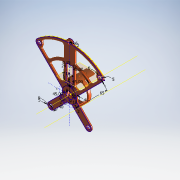
# Autodesk Inventor part: Pok Yaw Motor Face Mount
Saved by Autodesk Inventor 2018.2 (Build 222227000, 227)
## iProperties
Created: 2018-02-07
Part Number: Pok Yaw Motor Face Mount
Material: ABS Plastic
Document SubType Name: Modeling
Designer: Moochster
Density: 1.06 g/cm^3
Appearance: Smooth - Light Orange
Author: Moochster
Autodesk Inventor part; units mm, degrees
ref_plane "XZ Plane" through (0, 0, 0) normal (0, 1, 0) x (-1, 0, 0)
sketch "Sketch1" plane through (0, 0, 0) normal (0, 1, 0) x (-1, 0, 0)
  circle A0 centre (0, 0) radius 5 construction
  circle A1 centre (0, 0) radius 5.15
  circle A2 centre (8, 0) radius 1.25
  circle A3 centre (-8, 0) radius 1.25
  arc A4 (10.836268, 1.890843) -> (10.463737, 3.392669) centre (0, 0) ccw
  circle A5 centre (0, 0) radius 15 construction
  arc A6 (6.505618, 15.705952) -> (-6.505618, 15.705952) centre (0, 0) ccw
  arc A7 (5.740251, 13.858193) -> (-5.740251, 13.858193) centre (0, 0) ccw
  line L0 (6.505618, 15.705952) -> (5.740251, 13.858193)
  line L1 (-5.740251, 13.858193) -> (-6.505618, 15.705952)
  line L2 (3, 14.696938) -> (3, 10.583005)
  line L3 (-3, 14.696938) -> (-3, 10.583005)
  arc A8 (7.665151, -7.889579) -> (10.463737, -3.392669) centre (0, 0) ccw
  arc A9 (-7.665151, -7.889579) -> (-3.392669, -10.463737) centre (0, 0) ccw
  arc A10 (-10.665151, -2.693426) -> (-10.463737, -3.392669) centre (0, 0) ccw
  line L4 (5, 16.248077) -> (5, 28) construction
  line L5 (5, 28) -> (-5, 28) construction
  line L6 (-5, 28) -> (-5, 16.248077) construction
  line L7 (5.15, 16.201157) -> (5.15, 40.201157)
  line L8 (5.15, 40.201157) -> (-5.15, 40.201157)
  line L9 (-5.15, 40.201157) -> (-5.15, 16.201157)
  line L10 (0, 0) -> (28.284271, -28.284271) construction
  line L11 (0, 0) -> (33.023507, 0) construction
  circle A11 centre (28.284271, -28.284271) radius 3
  line L12 (3.392669, -10.463737) -> (6.464466, -13.535534)
  arc A12 (24.748737, -31.819805) -> (31.819805, -24.748737) centre (28.284271, -28.284271) ccw
  line L13 (31.819805, -24.748737) -> (15.024659, -7.953591)
  arc A13 (10.463737, -3.392669) -> (10.836268, 1.890843) centre (0, 0) ccw
  arc A14 (3.392669, -10.463737) -> (7.665151, -7.889579) centre (0, 0) ccw
  line L14 (0, 0) -> (0, -40.695352) construction
  circle A15 centre (-28.284271, -28.284271) radius 3
  line L15 (-3.392669, -10.463737) -> (-24.748737, -31.819805)
  arc A16 (-31.819805, -24.748737) -> (-24.748737, -31.819805) centre (-28.284271, -28.284271) ccw
  line L16 (-31.819805, -24.748737) -> (-10.463737, -3.392669)
  arc A17 (-10.463737, -3.392669) -> (-7.665151, -7.889579) centre (0, 0) ccw
  arc A18 (-3.392669, -10.463737) -> (3.392669, -10.463737) centre (0, 0) ccw
  arc A19 (-15.024659, -7.953591) -> (-7.953591, -15.024659) centre (0, 0) ccw
  arc A20 (7.953591, -15.024659) -> (15.024659, -7.953591) centre (0, 0) ccw
  arc A21 (6.464466, -13.535534) -> (13.535534, -6.464466) centre (0, 0) ccw
  arc A22 (-13.535534, -6.464466) -> (-6.464466, -13.535534) centre (0, 0) ccw
  line L17 (0, 0) -> (-45.961941, 45.961941) construction
  circle A23 centre (-45.961941, 45.961941) radius 3
  line L18 (-10.463737, 3.392669) -> (-49.497475, 42.426407)
  arc A24 (0, 68.107276) -> (-49.236593, 49.740386) centre (0, -7.071068) ccw
  line L19 (0, 0) -> (0, 68.107276) construction
  arc A25 (-49.236593, 49.740386) -> (-49.497475, 42.426407) centre (-45.961941, 45.961941) ccw
  arc A26 (-10.463737, 3.392669) -> (-10.665151, -2.693426) centre (0, 0) ccw
  circle A27 centre (45.961941, 45.961941) radius 3
  line L20 (10.463737, 3.392669) -> (49.497475, 42.426407)
  arc A28 (49.236593, 49.740386) -> (0, 68.107276) centre (0, -7.071068) ccw
  arc A29 (49.497475, 42.426407) -> (49.236593, 49.740386) centre (45.961941, 45.961941) ccw
  arc A30 (10.463737, 3.392669) -> (-10.463737, 3.392669) centre (0, 0) ccw
  line L21 (7.953591, -15.024659) -> (24.748737, -31.819805)
  line L22 (6.464466, -13.535534) -> (7.953591, -15.024659)
  line L23 (15.024659, -7.953591) -> (13.535534, -6.464466)
  line L24 (13.535534, -6.464466) -> (10.463737, -3.392669)
  point P0 (0, 17)
  point P1 (0, 28)
  point P2 (-53.159117, 46.088049)
  dimension "d0" = 10
  dimension "d1" = 0.15
  dimension "d2" = 2.5
  dimension "d4" = 8
  dimension "d5" = 8
  dimension "d6" = 22
  dimension "d10" = 4
  dimension "d14" = 2
  dimension "d15" = 6
  dimension "d16" = 45
  dimension "d47" = 10
  dimension "d48" = 11
  dimension "d56" = 0.15
  dimension "d57" = 0.15
  dimension "d58" = 24
  dimension "d61" = 45
  dimension "d62" = 40
  dimension "d63" = 5
  dimension "d64" = 6
  dimension "d65" = 2
  dimension "d66" = 2
  dimension "d69" = 45
  dimension "d70" = 65
  dimension "d71" = 6
  dimension "d72" = 5
  constraints: 63 point on circle, 50 end point, 31 centre point, 12 parallel, 11 symmetric about line, 11 tangent, 8 concentric, 8 point on line, 7 vertical, 4 coincident, 3 perpendicular, 2 horizontal alignment, 2 line through centre, 2 vertical alignment, 1 equal radius, 1 horizontal, 1 midpoint, 5 other
  measures "d0" diameter of A0
  measures "d1" radial gap between concentric circles of A0 A1
  measures "d2" diameter of A2
  measures "d4" distance of L10.start A2.centre
  measures "d5" distance of A3.centre L10.start
  measures "d6" diameter of A4
  measures "d10" radial gap between concentric circles of A4 A5
  measures "d14" radial gap between concentric circles of A6 A7
  measures "d15" distance between parallel lines of L2 L3
  measures "d16" angle of L0 L1
  measures "d47" distance of L4.end L5.end
  measures "d48" distance from line of point (0, 17) L5
  measures "d56" distance between parallel lines of L6 L9
  measures "d57" distance between parallel lines of L7 L4
  measures "d58" distance of L7.start L7.end
  measures "d61" angle of L10 L11
  measures "d62" distance of L10.start L10.end
  measures "d63" radius of A12
  measures "d64" diameter of A11
  measures "d65" radial gap between concentric circles of A19 A5
  measures "d66" radial gap between concentric circles of A21 A20
  measures "d69" angle of L17 L14
  measures "d70" distance of L17.start L17.end
  measures "d71" diameter of A23
  measures "d72" radius of A25
extrude "Extrusion1" add sketch "Sketch1" along normal blind 2 contours A13 A8 A14 A18 A9 A17 A10 A26 A30 A4 | A30 L2 A7 L0 A6 L7 L8 L9 L1 L3 L18 A25 A24 A28 A29 L20 | L24 A21 L12 A14 A8 | A30 L3 A7 L2 | L23 A20 L22 A21 | A7 L1 A6 L0 | L13 A12 L21 A20 | L15 A22 L16 A17 A9 | L15 A19 L16 A22 | L15 A16 L16 A19
extrude "Extrusion3" add sketch "Sketch1" along normal blind 32 contours A7 L1 A6 L0
extrude "Extrusion4" add sketch "Sketch1" along normal blind 16 contours L23 A20 L22 A21 | L15 A19 L16 A22
sketch "Sketch2" plane through (0, 0, 0) normal (1, 0, 0) x (0, 1, 0)
  line L0 (0, 17) -> (32, 17)
  line L1 (32, 15) -> (2, 15)
  line L2 (16, 15) -> (16, 17)
  line L3 (12, 15) -> (12, 17)
  line L4 (-6.4, 0) -> (38.4, 0)
  line L5 (16, -6.464466) -> (16, -13.535534)
  point P0 (0, 0)
  dimension "d25" = 4
  constraints: 4 end point, 3 point on line, 1 midpoint, 1 parallel, 1 vertical alignment
  measures "d25" distance between parallel lines of L2 L3
revolve "Revolution1" add sketch "Sketch2" angle 360 about axis through (0, -10, 0) along (0, 1, 0)
ref_plane "Work Plane1" through (0, 0, 17) normal (0, 0, 1) x (1, 0, 0)
sketch "Sketch3" plane through (0, 0, 17) normal (0, 0, 1) x (1, 0, 0)
  circle A0 centre (0, 8) radius 1.5
  circle A1 centre (0, 16) radius 1.5
  circle A2 centre (0, 24) radius 1.5
  point P0 (0, 0)
  point P1 (0, 0)
  point P2 (0, 0)
  dimension "d33" = 3
  dimension "d34" = 3
  dimension "d35" = 3
  dimension "d36" = 8
  dimension "d38" = 8
  dimension "d73" = 8
  constraints: 5 vertical alignment, 3 centre point
  measures "d33" diameter of A0
  measures "d34" diameter of A1
  measures "d35" diameter of A2
  measures "d36" distance of A0.centre A1.centre
  measures "d38" distance of A2.centre A1.centre
  measures "d73" distance of point (0, 0) A0.centre
extrude "Extrusion5" cut sketch "Sketch3" against normal up to surface round surface about axis through (0, 0, 0) along (0, 1, 0) radius 15 far side no
ref_plane "Work Plane4" through (12.020815, 0, -12.020815) normal (0.7071068, 0, -0.7071068) x (0, 1, 0)
ref_plane "Work Plane3" through (0, 0, 0) normal (0.7071068, 0, -0.7071068) x (0, 1, 0)
sketch "Sketch4" plane through (12.020815, 0, -12.020815) normal (0.7071068, 0, -0.7071068) x (0, 1, 0)
  circle A0 centre (12, 0) radius 1.5
  line L0 (0, -5) -> (0, 5) projected
  point P0 (0, 0)
  dimension "d44" = 3
  dimension "d68" = 12
  constraints: 1 centre point, 1 horizontal alignment, 1 midpoint
  measures "d44" diameter of A0
  measures "d68" distance from line of L0 A0.centre
extrude "Extrusion6" cut sketch "Sketch4" against normal up to next
mirror "Mirror1" about plane through (0, 0, 0) normal (1, 0, 0) of "Extrusion6"
sketch "Sketch7" plane through (0, 2, 0) normal (0, 1, 0) x (1, 0, 0)
  line L0 (8.15, -14.919031) -> (8.15, -40.201157)
  arc A0 (8.15, -14.919031) -> (13.35155, -10.523123) centre (0, 0) ccw
  arc A1 (8.15, -40.201157) -> (30.384505, -27.556078) centre (0, 0) ccw
  circle A2 centre (0, 0) radius 5.15
  line L1 (49.497475, -42.426407) -> (10.463737, -3.392669)
  line L2 (5.15, -16.201157) -> (5.15, -40.201157)
  arc A3 (-5.15, -16.201157) -> (5.15, -16.201157) centre (0, 0) ccw
  line L3 (13.35155, -10.523123) -> (30.384505, -27.556078)
  line L4 (8.15, -43.257911) -> (8.15, -64.645673)
  line L5 (32.508179, -29.679752) -> (44.135784, -41.307357)
  arc A4 (8.15, -64.645673) -> (43.663631, -50.402411) centre (0, 7.071068) ccw
  arc A5 (44.135784, -41.307357) -> (43.663631, -50.402411) centre (45.961941, -45.961941) ccw
  arc A6 (8.15, -43.257911) -> (32.508179, -29.679752) centre (0, 0) ccw
  circle A7 centre (45.961941, -45.961941) radius 3
  arc A8 (-49.236593, -49.740386) -> (49.236593, -49.740386) centre (0, 7.071068) ccw
  dimension "d74" = 3
  dimension "d75" = 3
  dimension "d76" = 3
  dimension "d77" = 3
  dimension "d78" = 2
  constraints: 10 point on circle, 8 end point, 6 concentric, 5 centre point, 2 vertical, 1 collinear, 1 horizontal alignment, 1 parallel, 1 vertical alignment
  measures "d74" distance between parallel lines of L2 L0
  measures "d75" distance between parallel lines of L1 L3
  measures "d76" radial gap between concentric circles of A1 A6
  measures "d77" radial gap between concentric circles of A8 A4
  measures "d78" radial gap between concentric circles of A7 A5
extrude "Extrusion8" cut sketch "Sketch7" against normal up to next contours A0 L3 A1 L0 | A6 L5 A5 A4 L4
fillet "Fillet4" radius 3 9 edges at (8.15, 1, 14.919) (13.3515, 1, 10.5231) (8.15, 1, 40.2012) (32.5082, 1, 29.6798) (30.3845, 1, 27.5561) (44.1358, 1, 41.3074) (43.6636, 1, 50.4024) (8.15, 1, 64.6457) (8.15, 1, 43.2579)
mirror "Mirror2" about plane through (0, 0, 0) normal (1, 0, 0) of "Fillet4", "Extrusion8"
sketch "Sketch8" plane through (0, 2, 0) normal (0, 1, 0) x (1, 0, 0)
  circle A0 centre (0, -68.107276) radius 3
  arc A1 (-49.236593, -49.740386) -> (49.236593, -49.740386) centre (0, 7.071068) ccw
  arc A2 (-4.997235, -67.941005) -> (4.997235, -67.941005) centre (0, -68.107276) ccw
  arc A3 (-4.997235, -67.941005) -> (-2.999403, -68.047419) centre (0, 7.071068) ccw
  arc A4 (-2.999403, -68.047419) -> (2.999403, -68.047419) centre (0, 7.071068) ccw
  arc A5 (2.999403, -68.047419) -> (4.997235, -67.941005) centre (0, 7.071068) ccw
  point P0 (0, 0)
  point P1 (0, -68.107276)
  dimension "d82" = 6
  dimension "d84" = 2
  constraints: 14 point on circle, 5 centre point, 2 concentric, 2 vertical alignment
  measures "d82" diameter of A0
  measures "d84" radial gap between concentric circles of A0 A2
extrude "Extrusion9" cut sketch "Sketch8" against normal up to next contours A0 A1 | A1 A0
extrude "Extrusion10" add sketch "Sketch8" against normal up to surface (2 mm away) contours A0 A1 A2
fillet "Fillet5" radius 3 2 edges at (4.9972, 1, 67.941) (-4.9972, 1, 67.941)
body "Solid1"
